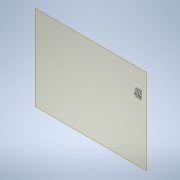
# Autodesk Inventor part: Extruder-Motherboard Cable Harness
Saved by Autodesk Inventor 2020 (Build 240168000, 168)
## iProperties
Created: 2019-12-22
Part Number: Extruder-Motherboard Cable Harness
Material: Generic
Document SubType Name: Modeling
Designer: pepd9
Density: 1 g/cm^3
Appearance: Default
Author: pepd9
Autodesk Inventor part; units mm, degrees
ref_plane "YZ Plane" through (0, 0, 0) normal (1, 0, 0) x (0, 1, 0)
ref_plane "XZ Plane" through (0, 0, 0) normal (0, 1, 0) x (-1, 0, 0)
ref_plane "XY Plane" through (0, 0, 0) normal (0, 0, 1) x (1, 0, 0)
ref_plane "Work Plane1" through (0, 0, 0) normal (0, 0, 1) x (1, 0, 0)
sketch "Sketch1" plane through (0, 0, 0) normal (0, 0, 1) x (1, 0, 0)
  circle A0 centre (228, 110.5) radius 1.1 construction
  circle A1 centre (239.5, 89) radius 1.1 construction
  line L0 (220, 118.5) -> (244.5, 118.5)
  line L1 (244.5, 118.5) -> (244.5, 81)
  line L2 (244.5, 81) -> (220, 81)
  line L3 (220, 81) -> (220, 118.5)
  point P0 (0, 0)
  dimension "d0" = 5
  dimension "d1" = 8
  dimension "d2" = 8
  dimension "d3" = 8
  constraints: 8 end point, 2 parallel, 1 horizontal, 1 perpendicular
  measures "d0" distance from line of A1.centre L1
  measures "d1" distance from line of L3 A0.centre
  measures "d2" distance from line of L2 A1.centre
  measures "d3" distance from line of L0 A0.centre
extrude "Extrusion1" add sketch "Sketch1" along normal blind 3
sketch "Sketch2" plane through (0, 0, 3) normal (0, 0, 1) x (1, 0, 0)
  circle A0 centre (228, 110.5) radius 1.1 projected
  circle A1 centre (239.5, 89) radius 1.1 projected
  point P0 (0, 0)
hole "Hole1" at (228, 110.5, 3) at (239.5, 89, 3) direction (0, 0, -1) diameter 3.4 end through all clearance for "Socket Head Cap Screw" size "M3" standard "Ansi Metric M Profile"
ref_plane "Work Plane2" through (220, 103.5, 0) normal (0, 1, 0) x (1, 0, 0)
sketch "Sketch3" plane through (220, 103.5, 0) normal (0, 1, 0) x (1, 0, 0)
  line L0 (0, -3) -> (24.5, -3) projected
  line L1 (12.25, -3) -> (12.25, -35.3077) construction
  circle A0 centre (12.25, -9) radius 5
  line L2 (24.5, -9) -> (24.5, -3)
  line L3 (7.25, -9) -> (0, -9)
  line L4 (0, -9) -> (0, -3)
  line L5 (0, -9) -> (24.5, -9)
  point P0 (-220, 0)
  point P1 (17.25, -9)
  dimension "d14" = 10
  dimension "d15" = 6
  dimension "d18" = 6
  constraints: 10 end point, 3 vertical, 2 horizontal, 1 horizontal alignment, 1 midpoint, 1 point on line, 3 other
  measures "d15" distance from line of L0 point (12.25, -9)
  measures "d18" distance of L3.end L0.start
extrude "Extrusion2" add sketch "Sketch3" against normal blind 8 contours L0 L2 L5 A0 L3 L4
sketch "Sketch4" plane through (237.25, 103.5, 9) normal (0, 0, 1) x (1, 0, 0)
  line L0 (-17.25, 0) -> (-10, 0) projected
  line L1 (-17.25, 0) -> (-17.25, -8) projected
  line L2 (-10, -8) -> (-17.25, -8) projected
  line L3 (-10, 0) -> (-10, -8) projected
  line L4 (0, 0) -> (7.25, 0) projected
  line L5 (0, 0) -> (0, -8) projected
  line L6 (7.25, -8) -> (0, -8) projected
  line L7 (7.25, 0) -> (7.25, -8) projected
  point P0 (-237.25, -103.5)
  point P1 (-13.625, -4)
  point P2 (3.625, -4)
hole "Hole2" at (223.625, 99.5, 9) at (240.875, 99.5, 9) direction (0, 0, -1) diameter 3.4 end through all clearance for "Socket Head Cap Screw" size "M3" standard "Ansi Metric M Profile"
sketch "Sketch5" plane through (0, 0, 0) normal (0, 0, -1) x (-1, 0, 0)
  circle A0 centre (-240.875, 99.5) radius 1.7 projected
  circle A1 centre (-223.625, 99.5) radius 1.7 projected
  line L0 (-243.625, 101.0877) -> (-240.875, 102.6754)
  line L1 (-240.875, 102.6754) -> (-238.125, 101.0877)
  line L2 (-238.125, 101.0877) -> (-238.125, 97.9123)
  line L3 (-238.125, 97.9123) -> (-240.875, 96.3246)
  line L4 (-240.875, 96.3246) -> (-243.625, 97.9123)
  line L5 (-243.625, 97.9123) -> (-243.625, 101.0877)
  line L6 (-226.375, 101.0877) -> (-223.625, 102.6754)
  line L7 (-223.625, 102.6754) -> (-220.875, 101.0877)
  line L8 (-220.875, 101.0877) -> (-220.875, 97.9123)
  line L9 (-220.875, 97.9123) -> (-223.625, 96.3246)
  line L10 (-223.625, 96.3246) -> (-226.375, 97.9123)
  line L11 (-226.375, 97.9123) -> (-226.375, 101.0877)
  point P0 (0, 0)
  dimension "d28" = 5.5
  dimension "d29" = 5.5
  constraints: 24 end point, 2 coincident, 26 other
  measures "d28" distance between parallel lines of L5 L2
  measures "d29" distance between parallel lines of L8 L11
extrude "Extrusion3" cut sketch "Sketch5" against normal blind 3
sketch "Sketch6" plane through (220, 103.5, 0) normal (0, 1, 0) x (1, 0, 0)
  line L0 (0, -3) -> (0, -9) projected
  line L1 (0, -9) -> (7.25, -9) projected
  arc A0 (17.25, -9) -> (7.25, -9) centre (12.25, -9) ccw projected
  line L2 (17.25, -9) -> (24.5, -9) projected
  line L3 (24.5, -9) -> (24.5, -3) projected
  line L4 (0, -3) -> (24.5, -3) projected
  line L5 (7.348, -8.015) -> (7.8461, -7.9714)
  line L6 (7.8461, -7.9714) -> (8.1881, -7.0317)
  line L7 (8.1881, -7.0317) -> (7.8051, -6.7103)
  point P0 (-220, 0)
  dimension "d32" = 5
  dimension "d33" = 45
  dimension "d34" = 115
  dimension "d35" = 1
  dimension "d36" = 0.5
  dimension "d37" = 0.5
  constraints: 6 end point, 2 point on circle
  measures "d32" angle of L5 L1
  measures "d33" angle of L5 L7
  measures "d34" angle of L6 L5
  measures "d35" distance of L5.end L6.end
  measures "d36" distance of L5.start L5.end
  measures "d37" distance of L6.end L7.end
extrude "Extrusion4" add sketch "Sketch6" against normal blind 1 contours A0 L7 L6 L5
pattern_circular "Circular Pattern1" count 5 over 140 about axis through (232.25, 103.5, 9) along (0, -1, 0) of "Extrusion4"
pattern_linear "Rectangular Pattern1" count 4 spacing 2.3 along (0, -1, 0) of "Extrusion4", "Circular Pattern1"
sketch "Sketch7" plane through (0, 0, 3) normal (0, 0, 1) x (1, 0, 0)
  line L0 (220, 103.5) -> (244.5, 103.5) projected
  line L1 (244.5, 103.5) -> (244.5, 118.5) projected
  line L2 (244.5, 118.5) -> (220, 118.5) projected
  line L3 (220, 118.5) -> (220, 103.5) projected
  circle A0 centre (228, 110.5) radius 1.7 projected
  circle A1 centre (239.5, 89) radius 1.7 projected
  line L4 (244.5, 95.5) -> (220, 95.5) projected
  line L5 (220, 95.5) -> (220, 81) projected
  line L6 (220, 81) -> (244.5, 81) projected
  line L7 (244.5, 81) -> (244.5, 95.5) projected
  circle A2 centre (228, 110.5) radius 1.7 projected
  circle A3 centre (228, 110.5) radius 3.5
  circle A4 centre (239.5, 89) radius 3.5
  line L8 (220, 118.5) -> (220, 103.5) projected
  line L9 (244.5, 103.5) -> (231.0594, 112.2)
  line L10 (224.9565, 112.2283) -> (220, 103.5)
  line L11 (244.5, 95.5) -> (220, 95.5) projected
  line L12 (220, 95.5) -> (237.844, 85.9166)
  line L13 (243, 89) -> (244.5, 95.5)
  point P0 (0, 0)
  dimension "d46" = 7
  dimension "d47" = 7
  constraints: 8 end point, 4 point on circle, 2 centre point, 2 coincident, 2 tangent
  measures "d46" diameter of A3
  measures "d47" diameter of A4
extrude "Extrusion5" cut sketch "Sketch7" against normal through all contours L3 L2 L1 L9 A3 L10 | L7 L6 L5 L12 A4 L13
fillet "Fillet1" radius 10 2 edges at (231.0594, 112.2, 1.5) (243, 89, 1.5)
fillet "Fillet2" radius 1 4 edges at (244.5, 103.5, 6) (244.5, 95.5, 6) (220, 95.5, 6) (220, 103.5, 6)
body "Solid1"
